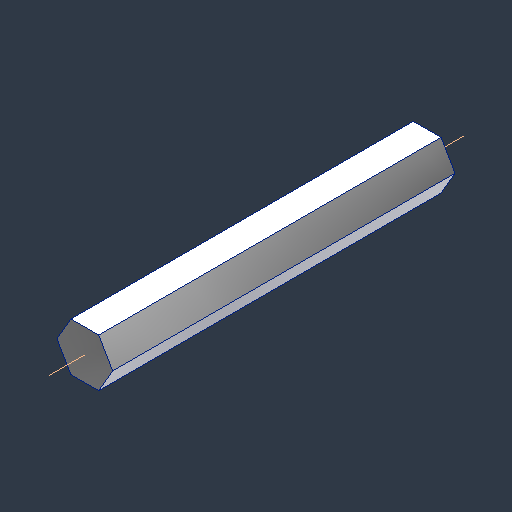
# Autodesk Inventor part: SHAFT,HEX,0.5,WHEELS,ARM
Saved by Autodesk Inventor 2024.3 (Build 283343000, 343)
## iProperties
ILogicPurgeVersion: 0.0.0.0
OnSaveVersion: 2.2.20.20
Category: _
Manager: _
Created: 2025-03-14
Part Number: SHAFT,HEX,0.5,WHEELS,ARM
Checked By: 00
Engr Approved By: _
User Status: Work In Process
Material: Aluminum 6061
Description: STANDARD (mm)
Document SubType Name: Modeling
Mfg Approved By: Stephen.Oerton
Designer: John Thibert
Manufacturer: Standard
Standards Organization: Custom
Density: 2.7 g/cm^3
Appearance: Aluminum - Flat
Mass: 34.0067 g
Surface Area: 42.4631 cm^2
Volume: 12.5951 cm^3
CN_MASS: 0
CN_SERVICEABLE: _
FIRST_DESCRIPTION: _
SECOND_DESCRIPTION: _
THIRD_DESCRIPTION: _
ModelCat: Uncategorized
Subject: _
Author: John Thibert
Keywords: -
Revision Number: A
Autodesk Inventor part; units mm, degrees
ref_plane "YZ Plane" through (0, 0, 0) normal (1, 0, 0) x (0, 1, 0)
ref_plane "XZ Plane" through (0, 0, 0) normal (0, 1, 0) x (-1, 0, 0)
ref_plane "XY Plane" through (0, 0, 0) normal (0, 0, 1) x (1, 0, 0)
sketch "Sketch2" plane through (0, 0, 0) normal (0, 0, 1) x (1, 0, 0)
  line L0 (3.6662, 6.35) -> (7.3323, 0)
  line L1 (7.3323, 0) -> (3.6662, -6.35)
  line L2 (3.6662, -6.35) -> (-3.6662, -6.35)
  line L3 (-3.6662, -6.35) -> (-7.3323, 0)
  line L4 (-7.3323, 0) -> (-3.6662, 6.35)
  line L5 (-3.6662, 6.35) -> (3.6662, 6.35)
  point P0 (0, 0)
  point P1 (0, 0)
  dimension "d0" = 12.7
  constraints: 12 end point, 1 coincident, 1 horizontal, 13 other
  measures "d0" distance between parallel lines of L2 L5
extrude "Extrusion1" add sketch "Sketch2" along normal mid plane 90.17
body "Solid1"
